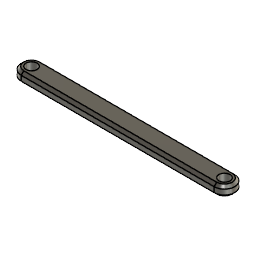
Support (Autodesk Fusion 360 design; units mm, degrees)
part number: 2026-04-04-04-06-12-103
Autodesk Fusion 360 part; units mm, degrees
sketch "Sketch1" plane through (0, 0, 0) normal (0, 0, 1) x (1, 0, 0)
  circle A0 centre (0, 0) radius 2.15
  circle A1 centre (0, 0) radius 4
  circle A2 centre (-74.481, 0) radius 2.15
  circle A3 centre (-74.481, 0) radius 4
  line L0 (0, 4) -> (-74.481, 4)
  line L1 (-74.481, -4) -> (0, -4)
  dimension "d1" = 4.3
  dimension "d2" = 8
  dimension "d3" = 74.481
  dimension "d4" = 4.3
  dimension "d5" = 8
  constraint coincident A0.centre A1.centre
  constraint concentric A0 A1
  constraint coincident A1 L0.start
  constraint concentric A2 A3
  constraint coincident A3 L0.end
  constraint tangent A3 L0
  constraint coincident A3 L1.start
  constraint coincident A1 L1.end
  constraint tangent A1 L1
  constraint horizontal L1
  measures "d1" diameter of A0
  measures "d2" diameter of A1
  measures "d3" distance of A0.centre A2.centre
  measures "d4" diameter of A2
  measures "d5" diameter of A3
extrude "Extrude1" add sketch "Sketch1" along normal blind 4
chamfer "Chamfer1" distance 1 angle 45 8 edges at (-37.2405, -4, 4) (4, 0, 4) (-37.2405, 4, 4) (-78.481, 0, 4) (-78.481, 0, 0) (-37.2405, -4, 0) (4, 0, 0) (-37.2405, 4, 0)
